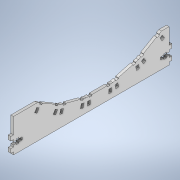
# Autodesk Inventor part: switchplate-support-04
Saved by Autodesk Inventor 2020.1 (Build 241239000, 239)
## iProperties
Created: 2019-06-27
Material: Acier, galvanisé
Document SubType Name: Modeling
Designer: Thibault
Density: 7.85 g/cm^3
Appearance: Aluminium - Poli
Mass: 11.7255 g
Surface Area: 33.7109 cm^2
Volume: 1.4937 cm^3
Part Number: switchplate-support-04
sa_0: 0.400 nd
height_shift: 0,000 mm
base_height: 25,000 mm
switchplate_depth: 121,000 mm
short_switchplate_depth: 87,585 mm
Author: Thibault
Autodesk Inventor part; units mm, degrees
ref_plane "YZ Plane" through (0, 0, 0) normal (1, 0, 0) x (0, 1, 0)
ref_plane "XZ Plane" through (0, 0, 0) normal (0, 1, 0) x (-1, 0, 0)
ref_plane "XY Plane" through (0, 0, 0) normal (0, 0, 1) x (1, 0, 0)
sketch "Anchor (screw side)" plane through (0, 0, 0) normal (0, 0, 1) x (1, 0, 0)
  circle A0 centre (93.7216, 50.3096) radius 1.05
  line L0 (91.2716, 51.3596) -> (88.1716, 51.3596)
  line L1 (88.1716, 51.3596) -> (88.1716, 49.2596)
  line L2 (88.1716, 49.2596) -> (91.2716, 49.2596)
  line L3 (91.2716, 49.2596) -> (91.2716, 51.3596)
  line L4 (99.2716, 51.3596) -> (96.1716, 51.3596)
  line L5 (96.1716, 51.3596) -> (96.1716, 49.2596)
  line L6 (96.1716, 49.2596) -> (99.2716, 49.2596)
  line L7 (99.2716, 49.2596) -> (99.2716, 51.3596)
  line L8 (91.2716, 51.3596) -> (96.1716, 49.2596) construction
  line L9 (96.1716, 51.3596) -> (91.2716, 49.2596) construction
  line L10 (86.1716, 53.3596) -> (101.2716, 53.3596) construction
  line L11 (101.2716, 53.3596) -> (101.2716, 47.2596) construction
  line L12 (101.2716, 47.2596) -> (86.1716, 47.2596) construction
  line L13 (86.1716, 47.2596) -> (86.1716, 53.3596) construction
  point P0 (103.5798, 50.1132)
  dimension "d27_1" = 2.1
  dimension "d28_1" = 3.1
  dimension "d29" = 2.1
  dimension "d32" = 4.9
  dimension "d34" = 2
  dimension "d35" = 2
  dimension "d36" = 2
  dimension "d37" = 2
  measures "d27_1" diameter of A0
  measures "d28_1" distance of L2.end L1.end
  measures "d29" distance of L1.end L0.end
  measures "d32" distance between parallel lines of L5 L3
  measures "d34" distance between parallel lines of L0 L10
  measures "d35" distance between parallel lines of L12 L2
  measures "d36" distance between parallel lines of L11 L7
  measures "d37" distance between parallel lines of L13 L1
sketch "Anchor (nut side)" plane through (0, 0, 0) normal (0, 0, 1) x (1, 0, 0)
  line L0 (10, 0) -> (8.55, 0)
  line L1 (8.55, 0) -> (8.55, -2)
  line L2 (8.55, -2) -> (9.35, -2)
  line L3 (9.35, -2) -> (9.35, -4)
  line L4 (5.65, -4) -> (5.65, -2)
  line L5 (5.65, -2) -> (6.45, -2)
  line L6 (6.45, -2) -> (6.45, 0)
  line L7 (6.45, 0) -> (5, 0)
  line L8 (2, 0) -> (2, 2)
  line L9 (2, 0) -> (3, 0) construction
  line L10 (2, 2) -> (5, 2)
  line L11 (5, 2) -> (5, 0)
  line L12 (10, 0) -> (10, 2)
  line L13 (10, 2) -> (13, 2)
  line L14 (13, 2) -> (13, 0)
  line L15 (0, 0) -> (2, 0)
  line L16 (13, 0) -> (15, 0)
  line L17 (5.65, -4) -> (6.45, -4)
  line L18 (9.35, -4) -> (8.55, -4)
  line L19 (6.45, -4) -> (6.45, -6.25)
  line L20 (8.55, -4) -> (8.55, -6.25)
  line L21 (6.7, -6.5) -> (7.5, -6.5)
  arc A0 (6.45, -6.25) -> (6.7, -6.5) centre (6.7, -6.25) ccw
  arc A1 (8.3, -6.5) -> (8.55, -6.25) centre (8.3, -6.25) ccw
  line L22 (7.5, -6.5) -> (8.3, -6.5)
  line L23 (7.5, -3.8983) -> (7.5, -9.959) construction
  point P0 (9.1321, -0.6227)
  point P1 (6.45, -6.5)
  point P2 (8.55, -6.5)
  dimension "d3" = 2
  dimension "d7" = 5
  dimension "d10" = 1.45
  dimension "d11" = 2
  dimension "d12" = 0.8
  dimension "d13" = 2
  dimension "d14" = 0.8
  dimension "d15" = 2.1
  dimension "d18" = 2
  dimension "d19" = 0.8
  dimension "d20" = 0.8
  dimension "d21" = 2.5
  dimension "d22" = 2.5
  dimension "d23" = 2.1
  dimension "d38" = 2
  dimension "d39" = 0.25
  dimension "d120" = 3
  measures "d3" distance of point (0, 0) L8.start
  measures "d7" distance of L7.end L0.start
  measures "d10" distance of L0.start L0.end
  measures "d11" distance of L0.end L1.end
  measures "d12" distance of L1.end L2.end
  measures "d13" distance of L2.end L3.end
  measures "d14" distance of L4.end L5.end
  measures "d15" distance of L6.end L0.end
  measures "d18" distance of L14.end point (15, 0)
  measures "d19" distance of L4.start L17.end
  measures "d20" distance of L3.end L18.end
  measures "d21" distance of L17.end point (6.45, -6.5)
  measures "d22" distance of L18.end point (8.55, -6.5)
  measures "d23" distance of L17.end L18.end
  measures "d38" distance of the line from the sketch origin of L10
  measures "d39" radius of A0
  measures "d120" distance of L8.end L10.end
sketch "Anchor (to 2ndary key support)" plane through (0, 0, 0) normal (0, 0, 1) x (1, 0, 0)
  line L0 (12.2429, 14.9506) -> (13.2929, 14.9506)
  line L1 (14.3429, 14.9506) -> (14.3429, 11.8506)
  line L2 (14.3429, 11.8506) -> (12.2429, 11.8506)
  line L3 (12.2429, 11.8506) -> (12.2429, 14.9506)
  line L4 (13.2929, 14.9506) -> (13.2929, 11.8506) construction
  line L5 (13.2929, 14.9506) -> (14.3429, 14.9506)
  point P0 (14.0267, 11.8837)
  dimension "d40" = 2.1
  dimension "d41" = 3.1
  measures "d40" distance of L1.end L2.end
  measures "d41" distance of L1.start L1.end
sketch "Switch support" plane through (0, 0, 0) normal (0, 0, 1) x (1, 0, 0)
  line L0 (14.375, 16.4474) -> (15.075, 16.4474)
  line L1 (15.075, 16.4474) -> (15.075, 15.6474)
  line L2 (15.075, 15.6474) -> (17.075, 15.6474)
  line L3 (17.075, 15.6474) -> (17.075, 16.4474)
  line L4 (17.075, 16.4474) -> (22.875, 16.4474)
  line L5 (28.675, 16.4474) -> (28.675, 15.6474)
  line L6 (28.675, 15.6474) -> (30.675, 15.6474)
  line L7 (30.675, 15.6474) -> (30.675, 16.4474)
  line L8 (30.675, 16.4474) -> (31.375, 16.4474)
  line L9 (22.875, 19.1721) -> (22.875, 15.8971) construction
  line L10 (22.875, 16.4474) -> (28.675, 16.4474)
  line L11 (13.775, 13.6474) -> (14.825, 13.6474)
  line L12 (15.875, 13.6474) -> (15.875, 10.5474)
  line L13 (15.875, 10.5474) -> (13.775, 10.5474)
  line L14 (13.775, 10.5474) -> (13.775, 13.6474)
  line L15 (14.825, 13.6474) -> (14.825, 10.5474) construction
  line L16 (14.825, 13.6474) -> (15.875, 13.6474)
  line L17 (29.875, 13.6474) -> (30.925, 13.6474)
  line L18 (31.975, 13.6474) -> (31.975, 10.5474)
  line L19 (31.975, 10.5474) -> (29.875, 10.5474)
  line L20 (29.875, 10.5474) -> (29.875, 13.6474)
  line L21 (30.925, 13.6474) -> (30.925, 10.5474) construction
  line L22 (30.925, 13.6474) -> (31.975, 13.6474)
  point P0 (20.0288, 26.7181)
  dimension "d43" = 0.8
  dimension "d44" = 2
  dimension "d45" = 11.6
  dimension "d46" = 2
  dimension "d47" = 0.7
  dimension "d48" = 17
  dimension "d51" = 2
  dimension "d121" = 8.05
  dimension "d123" = 8.05
  measures "d43" distance of L1.start L1.end
  measures "d44" distance of L1.end L2.end
  measures "d45" distance of L5.start L3.end
  measures "d46" distance of L5.end L6.end
  measures "d47" distance of L7.end point (31.375, 16.447)
  measures "d48" distance of point (31.375, 16.447) point (14.375, 16.447)
  measures "d51" length of L2
sketch "Sketch1" plane through (0, 0, 0) normal (1, 0, 0) x (0, 1, 0)
  line L0 (0, -121) -> (25, -121)
  line L1 (25, 0) -> (0, 0)
  line L2 (25, -121) -> (25, -113.278)
  line L3 (24.4162, -21.0111) -> (25, -20)
  line L4 (28.2121, -16.9724) -> (22.1003, -16.9724)
  line L5 (24.25, -21.299) -> (25, -20)
  line L6 (15.75, -36.0215) -> (15, -37.3205)
  line L7 (21.9473, -35.6102) -> (15.8356, -35.6102)
  line L8 (14.6118, -38.7694) -> (15, -37.3205)
  line L9 (10.2118, -55.1901) -> (9.8236, -56.639)
  line L10 (19.8511, -55.1756) -> (13.7394, -55.1756)
  line L11 (9.8236, -58.139) -> (9.8236, -56.639)
  line L12 (9.8236, -75.139) -> (9.8236, -76.639)
  line L13 (22.0358, -74.7409) -> (15.9241, -74.7409)
  line L14 (10.2118, -78.0879) -> (9.8236, -76.639)
  line L15 (14.6118, -94.5087) -> (15, -95.9575)
  line L16 (28.3566, -93.3787) -> (22.2449, -93.3787)
  line L17 (15.75, -97.2566) -> (15, -95.9575)
  line L18 (24.25, -111.979) -> (25, -113.278)
  line L19 (25, 0) -> (25, -20)
  line L20 (0, 0) -> (0, -121)
  line L21 (14.6118, -38.7694) -> (14.4306, -39.4455)
  line L22 (14.4306, -39.4455) -> (13.6579, -39.2385)
  line L23 (13.6579, -39.2385) -> (13.1402, -41.1703)
  line L24 (13.1402, -41.1703) -> (13.913, -41.3774)
  line L25 (13.913, -41.3774) -> (12.4118, -46.9798)
  line L26 (10.9107, -52.5821) -> (10.1379, -52.3751)
  line L27 (10.1379, -52.3751) -> (9.6203, -54.3069)
  line L28 (9.6203, -54.3069) -> (10.393, -54.514)
  line L29 (10.393, -54.514) -> (10.2118, -55.1901)
  line L30 (15.0436, -47.685) -> (11.8802, -46.8373) construction
  line L31 (12.4118, -46.9798) -> (10.9107, -52.5821)
  line L32 (12.0625, -37.4651) -> (11.7907, -38.4794)
  line L33 (11.519, -39.4936) -> (8.5246, -38.6913)
  line L34 (8.5246, -38.6913) -> (9.0681, -36.6628)
  line L35 (9.0681, -36.6628) -> (12.0625, -37.4651)
  line L36 (11.7907, -38.4794) -> (8.7963, -37.677) construction
  line L37 (11.7907, -38.4794) -> (11.519, -39.4936)
  line L38 (7.8955, -53.0166) -> (7.6237, -54.0308)
  line L39 (7.352, -55.045) -> (4.3576, -54.2427)
  line L40 (4.3576, -54.2427) -> (4.9011, -52.2142)
  line L41 (4.9011, -52.2142) -> (7.8955, -53.0166)
  line L42 (7.6237, -54.0308) -> (4.6294, -53.2284) construction
  line L43 (7.6237, -54.0308) -> (7.352, -55.045)
  line L44 (24.25, -21.299) -> (23.9, -21.9053)
  line L45 (23.9, -21.9053) -> (23.2072, -21.5053)
  line L46 (23.2072, -21.5053) -> (22.2072, -23.2373)
  line L47 (22.2072, -23.2373) -> (22.9, -23.6373)
  line L48 (22.9, -23.6373) -> (20, -28.6603)
  line L49 (17.1, -33.6832) -> (16.4072, -33.2832)
  line L50 (16.4072, -33.2832) -> (15.4072, -35.0153)
  line L51 (15.4072, -35.0153) -> (16.1, -35.4153)
  line L52 (16.1, -35.4153) -> (15.75, -36.0215)
  line L53 (22.3596, -30.0226) -> (19.5234, -28.3851) construction
  line L54 (20, -28.6603) -> (17.1, -33.6832)
  line L55 (22.1251, -19.3794) -> (21.6001, -20.2887)
  line L56 (21.0751, -21.1981) -> (18.3905, -19.6481)
  line L57 (18.3905, -19.6481) -> (19.4405, -17.8294)
  line L58 (19.4405, -17.8294) -> (22.1251, -19.3794)
  line L59 (21.6001, -20.2887) -> (18.9155, -18.7387) construction
  line L60 (21.6001, -20.2887) -> (21.0751, -21.1981)
  line L61 (14.0751, -33.3224) -> (13.5501, -34.2318)
  line L62 (13.0251, -35.1411) -> (10.3405, -33.5911)
  line L63 (10.3405, -33.5911) -> (11.3905, -31.7724)
  line L64 (11.3905, -31.7724) -> (14.0751, -33.3224)
  line L65 (13.5501, -34.2318) -> (10.8655, -32.6818) construction
  line L66 (13.5501, -34.2318) -> (13.0251, -35.1411)
  line L67 (9.8236, -58.139) -> (9.8236, -58.839)
  line L68 (9.8236, -58.839) -> (9.0236, -58.839)
  line L69 (9.0236, -58.839) -> (9.0236, -60.839)
  line L70 (9.0236, -60.839) -> (9.8236, -60.839)
  line L71 (9.8236, -60.839) -> (9.8236, -66.639)
  line L72 (9.8236, -72.439) -> (9.0236, -72.439)
  line L73 (9.0236, -72.439) -> (9.0236, -74.439)
  line L74 (9.0236, -74.439) -> (9.8236, -74.439)
  line L75 (9.8236, -74.439) -> (9.8236, -75.139)
  line L76 (12.5483, -66.639) -> (9.2733, -66.639) construction
  line L77 (9.8236, -66.639) -> (9.8236, -72.439)
  line L78 (7.0236, -57.539) -> (7.0236, -58.589)
  line L79 (7.0236, -59.639) -> (3.9236, -59.639)
  line L80 (3.9236, -59.639) -> (3.9236, -57.539)
  line L81 (3.9236, -57.539) -> (7.0236, -57.539)
  line L82 (7.0236, -58.589) -> (3.9236, -58.589) construction
  line L83 (7.0236, -58.589) -> (7.0236, -59.639)
  line L84 (7.0236, -73.639) -> (7.0236, -74.689)
  line L85 (7.0236, -75.739) -> (3.9236, -75.739)
  line L86 (3.9236, -75.739) -> (3.9236, -73.639)
  line L87 (3.9236, -73.639) -> (7.0236, -73.639)
  line L88 (7.0236, -74.689) -> (3.9236, -74.689) construction
  line L89 (7.0236, -74.689) -> (7.0236, -75.739)
  line L90 (10.2118, -78.0879) -> (10.393, -78.7641)
  line L91 (10.393, -78.7641) -> (9.6203, -78.9711)
  line L92 (9.6203, -78.9711) -> (10.1379, -80.903)
  line L93 (10.1379, -80.903) -> (10.9107, -80.6959)
  line L94 (10.9107, -80.6959) -> (12.4118, -86.2983)
  line L95 (13.913, -91.9007) -> (13.1402, -92.1077)
  line L96 (13.1402, -92.1077) -> (13.6579, -94.0396)
  line L97 (13.6579, -94.0396) -> (14.4306, -93.8325)
  line L98 (14.4306, -93.8325) -> (14.6118, -94.5087)
  line L99 (15.0436, -85.5931) -> (11.8802, -86.4407) construction
  line L100 (12.4118, -86.2983) -> (13.913, -91.9007)
  line L101 (7.352, -78.2331) -> (7.6237, -79.2473)
  line L102 (7.8955, -80.2615) -> (4.9011, -81.0638)
  line L103 (4.9011, -81.0638) -> (4.3576, -79.0354)
  line L104 (4.3576, -79.0354) -> (7.352, -78.2331)
  line L105 (7.6237, -79.2473) -> (4.6294, -80.0496) construction
  line L106 (7.6237, -79.2473) -> (7.8955, -80.2615)
  line L107 (11.519, -93.7845) -> (11.7907, -94.7987)
  line L108 (12.0625, -95.8129) -> (9.0681, -96.6152)
  line L109 (9.0681, -96.6152) -> (8.5246, -94.5868)
  line L110 (8.5246, -94.5868) -> (11.519, -93.7845)
  line L111 (11.7907, -94.7987) -> (8.7963, -95.601) construction
  line L112 (11.7907, -94.7987) -> (12.0625, -95.8129)
  line L113 (15.75, -97.2566) -> (16.1, -97.8628)
  line L114 (16.1, -97.8628) -> (15.4072, -98.2628)
  line L115 (15.4072, -98.2628) -> (16.4072, -99.9948)
  line L116 (16.4072, -99.9948) -> (17.1, -99.5948)
  line L117 (17.1, -99.5948) -> (20, -104.6178)
  line L118 (22.9, -109.6407) -> (22.2072, -110.0407)
  line L119 (22.2072, -110.0407) -> (23.2072, -111.7728)
  line L120 (23.2072, -111.7728) -> (23.9, -111.3728)
  line L121 (23.9, -111.3728) -> (24.25, -111.979)
  line L122 (22.3596, -103.2555) -> (19.5234, -104.893) construction
  line L123 (20, -104.6178) -> (22.9, -109.6407)
  line L124 (13.0251, -98.137) -> (13.5501, -99.0463)
  line L125 (14.0751, -99.9556) -> (11.3905, -101.5056)
  line L126 (11.3905, -101.5056) -> (10.3405, -99.687)
  line L127 (10.3405, -99.687) -> (13.0251, -98.137)
  line L128 (13.5501, -99.0463) -> (10.8655, -100.5963) construction
  line L129 (13.5501, -99.0463) -> (14.0751, -99.9556)
  line L130 (21.0751, -112.08) -> (21.6001, -112.9893)
  line L131 (22.1251, -113.8986) -> (19.4405, -115.4486)
  line L132 (19.4405, -115.4486) -> (18.3905, -113.63)
  line L133 (18.3905, -113.63) -> (21.0751, -112.08)
  line L134 (21.6001, -112.9893) -> (18.9155, -114.5393) construction
  line L135 (21.6001, -112.9893) -> (22.1251, -113.8986)
  point P0 (24.25, -111.979)
  point P1 (14.6118, -94.5087)
  point P2 (10.2118, -78.0879)
  point P3 (10.2118, -55.1901)
  point P4 (14.6118, -38.7694)
  point P5 (24.25, -21.299)
  dimension "height" = 25
  dimension "d193" = 25
  dimension "k1_a" = 1.5
  dimension "k1_b" = 1.5
  dimension "k2_a" = 1.5
  dimension "k2_b" = 1.5
  dimension "k3_a" = 1.5
  dimension "k3_b" = 1.5
  dimension "k4_a" = 1.5
  dimension "k4_b" = 1.5
  dimension "k5_a" = 1.5
  dimension "k5_b" = 1.5
  dimension "d257" = 20
  dimension "k1_angle" = 120
  dimension "k2_angle" = 105
  dimension "k3_angle" = 90
  dimension "k4_angle" = 75
  dimension "k5_angle" = 60
  constraints: 42 end point, 7 horizontal, 4 vertical, 1 collinear, 1 vertical alignment, 19 other
  measures "height" distance of L1.start L1.end
  measures "d193" distance of L0.end L0.start
  measures "k1_a" distance of L3.end L5.start
  measures "k1_b" distance of L6.end L6.start
  measures "k2_a" distance of L8.start L6.end
  measures "k2_b" distance of L9.end L9.start
  measures "k3_a" distance of L11.start L9.end
  measures "k3_b" distance of L12.end L12.start
  measures "k4_a" distance of L14.start L12.end
  measures "k4_b" distance of L15.end L15.start
  measures "k5_a" distance of L17.start L15.end
  measures "k5_b" distance of L2.end L18.start
  measures "d257" distance of L1.start L3.end
  measures "k3_angle" angle to the sketch y axis of L10
extrude "Base" add sketch "Sketch1" along normal blind 2
sketch "Sketch2" plane through (0, 0, 0) normal (-1, 0, 0) x (0, 0, 1)
  line L0 (-189.6233, 19.237) -> (-189.6233, -29.346)
  line L1 (129.5944, 112.7524) -> (129.5944, -29.346)
  line L2 (129.5944, -29.346) -> (-189.6233, -29.346)
  line L3 (-119, 15) -> (-119, 103.8044)
  line L4 (-119, 103.8044) -> (-189.6233, 103.8044)
  line L5 (-189.6233, 103.8044) -> (-189.6233, 19.237)
  line L6 (-2, 15) -> (-2, 112.7524)
  line L7 (-2, 112.7524) -> (129.5944, 112.7524)
  line L8 (-121, 0) -> (-121, 25) projected
  line L9 (0, 25) -> (0, 0) projected
  line L10 (-119, -2) -> (-2, -2)
  line L11 (-96.1009, -2) -> (-99.1009, -2) projected
  line L12 (-119, 0) -> (-119, -2)
  line L13 (-2, 0) -> (-2, -2)
  line L14 (-119, 10) -> (-119, 8.55)
  line L15 (-119, 8.55) -> (-117, 8.55)
  line L16 (-117, 8.55) -> (-117, 9.35)
  line L17 (-117, 9.35) -> (-115, 9.35)
  line L18 (-115, 5.65) -> (-117, 5.65)
  line L19 (-117, 5.65) -> (-117, 6.45)
  line L20 (-117, 6.45) -> (-119, 6.45)
  line L21 (-119, 6.45) -> (-119, 5)
  line L22 (-119, 2) -> (-121, 2)
  line L23 (-119, 2) -> (-119, 3) construction
  line L24 (-121, 2) -> (-121, 5)
  line L25 (-121, 5) -> (-119, 5)
  line L26 (-119, 10) -> (-121, 10)
  line L27 (-121, 10) -> (-121, 13)
  line L28 (-121, 13) -> (-119, 13)
  line L29 (-119, 0) -> (-119, 2)
  line L30 (-119, 13) -> (-119, 15)
  line L31 (-115, 5.65) -> (-115, 6.45)
  line L32 (-115, 9.35) -> (-115, 8.55)
  line L33 (-115, 6.45) -> (-112.75, 6.45)
  line L34 (-115, 8.55) -> (-112.75, 8.55)
  line L35 (-112.5, 6.7) -> (-112.5, 7.5)
  arc A0 (-112.75, 6.45) -> (-112.5, 6.7) centre (-112.75, 6.7) ccw
  arc A1 (-112.5, 8.3) -> (-112.75, 8.55) centre (-112.75, 8.3) ccw
  line L36 (-112.5, 7.5) -> (-112.5, 8.3)
  line L37 (-115.1017, 7.5) -> (-109.041, 7.5) construction
  line L38 (-2, 5) -> (-2, 6.45)
  line L39 (-2, 6.45) -> (-4, 6.45)
  line L40 (-4, 6.45) -> (-4, 5.65)
  line L41 (-4, 5.65) -> (-6, 5.65)
  line L42 (-6, 9.35) -> (-4, 9.35)
  line L43 (-4, 9.35) -> (-4, 8.55)
  line L44 (-4, 8.55) -> (-2, 8.55)
  line L45 (-2, 8.55) -> (-2, 10)
  line L46 (-2, 13) -> (0, 13)
  line L47 (-2, 13) -> (-2, 12) construction
  line L48 (0, 13) -> (0, 10)
  line L49 (0, 10) -> (-2, 10)
  line L50 (-2, 5) -> (0, 5)
  line L51 (0, 5) -> (0, 2)
  line L52 (0, 2) -> (-2, 2)
  line L53 (-2, 15) -> (-2, 13)
  line L54 (-2, 2) -> (-2, 0)
  line L55 (-6, 9.35) -> (-6, 8.55)
  line L56 (-6, 5.65) -> (-6, 6.45)
  line L57 (-6, 8.55) -> (-8.25, 8.55)
  line L58 (-6, 6.45) -> (-8.25, 6.45)
  line L59 (-8.5, 8.3) -> (-8.5, 7.5)
  arc A2 (-8.25, 8.55) -> (-8.5, 8.3) centre (-8.25, 8.3) ccw
  arc A3 (-8.5, 6.7) -> (-8.25, 6.45) centre (-8.25, 6.7) ccw
  line L60 (-8.5, 7.5) -> (-8.5, 6.7)
  line L61 (-5.8983, 7.5) -> (-11.959, 7.5) construction
  point P0 (110, 20)
  point P1 (-121, 0)
  point P2 (0, 35.5246)
  constraints: 22 end point, 5 vertical, 2 horizontal, 2 parallel, 1 collinear, 1 perpendicular, 7 other
extrude "Standard anchors" cut sketch "Sketch2" against normal through all
sketch "Esquisse7" plane through (0, 0, 0) normal (-1, 0, 0) x (0, 0, 1)
  line L0 (-104.5, 8.35) -> (-102.5, 8.35) construction
  line L1 (-106.5, 9.15) -> (-104.5, 9.15) construction
  line L2 (-104.5, 5.85) -> (-106.5, 5.85) construction
  line L3 (-102.5, 6.65) -> (-104.5, 6.65) construction
  line L4 (-109, 9.15) -> (-100.5, 9.15)
  line L5 (-109, 5.85) -> (-100.5, 5.85)
  line L6 (-109, 10) -> (-109, 8.35) construction
  line L7 (-109, 9.15) -> (-109, 5.85)
  arc A0 (-102.5, 6.65) -> (-102.5, 8.35) centre (-102.5, 7.5) ccw projected
  line L8 (-100.5, 5.85) -> (-100.5, 9.15)
  point P0 (1.5, 20)
  point P1 (108.5, 20)
  point P2 (108.5, 0)
  point P3 (1.5, 0)
  point P4 (-2, 10)
  point P5 (-2, 5)
  point P6 (7.6691, 10.85)
  point P7 (8.8147, 9.7576)
  point P8 (-111, 0)
  point P9 (-102.77, 8.35)
  point P10 (-100.7609, 7.9198)
  dimension "d203" = 2
  constraints: 8 end point, 2 collinear, 1 perpendicular, 1 vertical, 2 other
  measures "d203" distance from line of L8 A0.centre
extrude "No back screw hole" [suppressed]
sketch "Esquisse13" plane through (2, 0, 0) normal (1, 0, 0) x (0, 0, -1)
  line L0 (31.7724, 11.3905) -> (33.3224, 14.0751)
  line L1 (33.3224, 14.0751) -> (35.1411, 13.0251)
  line L2 (35.1411, 13.0251) -> (33.5911, 10.3405)
  line L3 (33.5911, 10.3405) -> (31.7724, 11.3905)
  line L4 (35.1411, 13.0251) -> (33.5911, 10.3405) projected
  line L5 (31.7724, 11.3905) -> (33.3224, 14.0751) projected
  line L6 (33.3224, 14.0751) -> (35.1411, 13.0251) projected
  line L7 (33.5911, 10.3405) -> (31.7724, 11.3905) projected
  point P0 (0, 0)
  constraints: 8 end point, 4 collinear
extrude "Hole fixup" [suppressed]
sketch "Esquisse8" plane through (0, 0, 0) normal (-1, 0, 0) x (0, 0, 1)
  line L0 (0, 0) -> (-100.5509, 0) projected
  line L1 (0, 0) -> (-20.4545, 0)
  line L2 (0, 63.8513) -> (0, 0)
  line L3 (0, 25) -> (0, 0) projected
  line L4 (-35.4153, 63.8513) -> (0, 63.8513)
  line L5 (-35.4153, 63.8513) -> (-35.4153, 15)
  line L6 (-121, 2) -> (-121, 25) projected
  line L7 (-35.4153, 5) -> (-35.4153, 6.45)
  line L8 (-35.4153, 6.45) -> (-37.4153, 6.45)
  line L9 (-37.4153, 6.45) -> (-37.4153, 5.65)
  line L10 (-37.4153, 5.65) -> (-39.4153, 5.65)
  line L11 (-39.4153, 9.35) -> (-37.4153, 9.35)
  line L12 (-37.4153, 9.35) -> (-37.4153, 8.55)
  line L13 (-37.4153, 8.55) -> (-35.4153, 8.55)
  line L14 (-35.4153, 8.55) -> (-35.4153, 10)
  line L15 (-35.4153, 13) -> (-33.4153, 13)
  line L16 (-35.4153, 13) -> (-35.4153, 12) construction
  line L17 (-33.4153, 13) -> (-33.4153, 10)
  line L18 (-33.4153, 10) -> (-35.4153, 10)
  line L19 (-35.4153, 5) -> (-33.4153, 5)
  line L20 (-33.4153, 5) -> (-33.4153, 2)
  line L21 (-33.4153, 2) -> (-35.4153, 2)
  line L22 (-35.4153, 15) -> (-35.4153, 13)
  line L23 (-35.4153, 2) -> (-35.4153, 0)
  line L24 (-39.4153, 9.35) -> (-39.4153, 8.55)
  line L25 (-39.4153, 5.65) -> (-39.4153, 6.45)
  line L26 (-39.4153, 8.55) -> (-41.6653, 8.55)
  line L27 (-39.4153, 6.45) -> (-41.6653, 6.45)
  line L28 (-41.9153, 8.3) -> (-41.9153, 7.5)
  arc A0 (-41.6653, 8.55) -> (-41.9153, 8.3) centre (-41.6653, 8.3) ccw
  arc A1 (-41.9153, 6.7) -> (-41.6653, 6.45) centre (-41.6653, 6.7) ccw
  line L29 (-41.9153, 7.5) -> (-41.9153, 6.7)
  line L30 (-39.3135, 7.5) -> (-45.3743, 7.5) construction
  point P0 (110, 0)
  point P1 (-109, 0)
  point P2 (-121, 0)
  point P3 (0, 12.75)
  point P4 (0, 10.25)
  point P5 (0, 12)
  point P6 (-35.4153, 16.1)
  point P7 (-35.4153, 15)
  point P8 (-35.4153, 0)
  point P9 (-121, 5)
  dimension "d232" = 20.4545
  constraints: 8 end point, 3 vertical, 2 collinear, 2 horizontal, 1 parallel, 1 point on line, 1 other
  measures "d232" distance of L0.start L1.end
extrude "Short plate" [suppressed]
derived "shared_parameters.ipt"
equation "\"depth_shift\" = 14"
equation "\"angle\" = 15deg"
equation "\"a_default\" = 1.5"
equation "\"b_default\" = 1.5"
